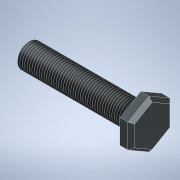
# Autodesk Inventor part: bolt
Saved by Autodesk Inventor 2021 (Build 250183000, 183)
## iProperties
Created: 2021-07-14
Part Number: bolt
Material: Iron, Cast
Document SubType Name: Modeling
Designer: HP
Density: 7.15 g/cm^3
Appearance: Iron Gray
Author: HP
Autodesk Inventor part; units mm, degrees
ref_plane "YZ Plane" through (0, 0, 0) normal (1, 0, 0) x (0, 1, 0)
ref_plane "XZ Plane" through (0, 0, 0) normal (0, 1, 0) x (-1, 0, 0)
ref_plane "XY Plane" through (0, 0, 0) normal (0, 0, 1) x (1, 0, 0)
sketch "Sketch1" plane through (0, 0, 0) normal (1, 0, 0) x (0, 1, 0)
  circle A0 centre (0, 0) radius 7.45
  dimension "d0" = 14.9
  constraints: 1 centre point, 1 coincident
  measures "d0" diameter of A0
extrude "Extrusion1" add sketch "Sketch1" along normal blind 70
sketch "Sketch2" plane through (70, 0, 0) normal (1, 0, 0) x (0, 0, -1)
  line L0 (0, 14.962) -> (12.9575, 7.481)
  line L1 (12.9575, 7.481) -> (12.9575, -7.481)
  line L2 (12.9575, -7.481) -> (0, -14.962)
  line L3 (0, -14.962) -> (-12.9575, -7.481)
  line L4 (-12.9575, -7.481) -> (-12.9575, 7.481)
  line L5 (-12.9575, 7.481) -> (0, 14.962)
  point P0 (0, 0)
  point P1 (0, 0)
  dimension "d12" = 25.915
  dimension "d13" = 14.962
  constraints: 12 end point, 1 coincident, 13 other
  measures "d12" distance between parallel lines of L1 L4
  measures "d13" distance of L3.end L4.end
extrude "Extrusion2" add sketch "Sketch2" along normal blind 7
chamfer "Chamfer1" distance 1 angle 45 1 edges at (0, -7.45, 0)
sketch "Sketch3" plane through (0, 0, 0) normal (0, 0, 1) x (1, 0, 0)
  point P0 (0, 0)
thread "Thread2" size "M15x1.5" class "6g" standard "ANSI Metric M Profile" full length
chamfer "Chamfer2" distance 2 angle 45 6 edges at (77, 11.2215, -6.4788) (77, 11.2215, 6.4788) (77, 0, 12.9575) (77, -11.2215, 6.4788) (77, -11.2215, -6.4788) (77, 0, -12.9575)
body "Solid1"
